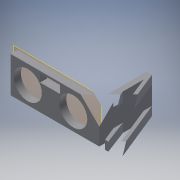
# Autodesk Inventor part: USsensor holder
Saved by Autodesk Inventor 2016 (Build 200138000, 138)
## iProperties
Created: 2018-11-07
Part Number: USsensor holder
Material: Generic
Document SubType Name: Modeling
Designer: anjal
Density: 1 g/cm^3
Appearance: Default
Author: anjal
Autodesk Inventor part; units mm, degrees
ref_plane "YZ Plane" through (0, 0, 0) normal (1, 0, 0) x (0, 1, 0)
ref_plane "XZ Plane" through (0, 0, 0) normal (0, 1, 0) x (-1, 0, 0)
ref_plane "XY Plane" through (0, 0, 0) normal (0, 0, 1) x (1, 0, 0)
ref_plane "Work Plane1" through (7.2648, 18.7113, 1.7167) normal (0, 0, 1) x (1, 0, 0)
sketch "Sketch1" plane through (7.2648, 18.7113, 1.7167) normal (0, 0, 1) x (1, 0, 0)
  circle A0 centre (-12.9413, -0.2667) radius 7.9502 projected
  line L0 (-5.933, 4.5118) -> (5.37, 4.5118) projected
  line L1 (5.37, 9.0584) -> (-5.933, 9.0584) projected
  line L2 (5.37, 9.0584) -> (-5.933, 9.0584) projected
  circle A1 centre (-12.9413, -0.2667) radius 7.9502 projected
  circle A2 centre (12.9413, -0.2667) radius 7.9502 projected
  line L3 (22.7457, -10.1981) -> (22.7457, 10.1981)
  line L4 (22.7457, 10.1981) -> (-22.7457, 10.1981) projected
  line L5 (-22.7457, -10.1981) -> (22.7457, -10.1981)
  line L6 (-22.7457, 10.1981) -> (-22.7457, -10.1981)
  line L7 (-5.933, 6.444) -> (-5.933, 4.5118) projected
  line L8 (-5.933, 9.0584) -> (-5.933, 7.1262) projected
  line L9 (5.37, 4.5118) -> (5.37, 9.0584)
  line L10 (-5.933, 9.0584) -> (-5.933, 4.5118)
  circle A3 centre (-12.9413, -0.2667) radius 8.25
  circle A4 centre (12.9413, -0.2667) radius 8.25
  point P0 (-7.2648, -18.7113)
  dimension "d5" = 16.5
  dimension "d6" = 16.5
  constraints: 10 end point, 3 vertical, 2 centre point, 2 coincident, 1 horizontal, 1 parallel, 3 other
  measures "d5" diameter of A3
  measures "d6" diameter of A4
extrude "Extrusion1" add sketch "Sketch1" along normal blind 4 contours L5 L6 L4 L3 | A3 | A4
sketch "Sketch2" plane through (7.2648, 18.7113, 5.7167) normal (0, 0, 1) x (1, 0, 0)
  line L0 (22.7457, -10.1981) -> (22.7457, 10.1981)
  line L1 (22.7457, 10.1981) -> (27.7457, 10.1981)
  line L2 (27.7457, 10.1981) -> (27.7457, -10.1981)
  line L3 (27.7457, -10.1981) -> (22.7457, -10.1981)
  line L4 (22.7457, -10.1981) -> (22.7457, 10.1981)
  line L5 (24.7457, 10.1981) -> (24.7457, -10.1981)
  point P0 (-7.2648, -18.7113)
  dimension "d7" = 5
  dimension "d8" = 2
  constraints: 12 end point, 2 parallel, 2 perpendicular, 2 point on line, 1 horizontal
  measures "d7" distance of L0.end L1.end
  measures "d8" distance between parallel lines of L0 L5
extrude "Extrusion3" add sketch "Sketch2" against normal blind 30 contours L5 L1 L2 L3
sketch "Sketch3" plane through (7.2648, 18.7113, 5.7167) normal (0, 0, 1) x (1, 0, 0)
  line L0 (22.7457, -10.1981) -> (22.7457, 10.1981) projected
  line L1 (24.7457, -10.1981) -> (24.7457, 10.1981) projected
  line L2 (22.7457, 10.1981) -> (24.7457, 10.1981)
  line L3 (24.7457, 10.1981) -> (24.7457, -10.1981)
  line L4 (24.7457, -10.1981) -> (22.7457, -10.1981)
  line L5 (22.7457, -10.1981) -> (22.7457, 10.1981)
  point P0 (-7.2648, -18.7113)
  constraints: 8 end point, 2 parallel, 1 horizontal, 1 perpendicular
extrude "Extrusion4" add sketch "Sketch3" against normal blind 4
sketch "Sketch4" plane through (-15.4809, 28.9094, 5.7167) normal (0, 1, 0) x (1, 0, 0)
  line L0 (50.4914, 0) -> (50.4914, 30) projected
  line L1 (50.4914, 30) -> (62.668, 0)
  line L2 (62.668, 0) -> (60.736, 0)
  line L3 (60.736, 0) -> (50.4914, 25.24)
  line L4 (55.6137, 0) -> (50.4914, 13.4027)
  line L5 (53.764, 0) -> (50.4914, 8.0628)
  line L6 (50.4914, 13.4027) -> (50.4914, 8.0628)
  line L7 (53.764, 0) -> (55.6137, 0)
  point P0 (15.4809, 5.7167)
  constraints: 14 end point, 5 point on line, 2 parallel, 2 perpendicular, 1 collinear
extrude "Extrusion5" add sketch "Sketch4" against normal blind 5
sketch "Sketch5" plane through (-15.4809, 8.5132, 1.7167) normal (0, -1, 0) x (1, 0, 0)
  line L0 (50.4914, -26) -> (50.4914, -21.24) projected
  line L1 (50.4914, -26) -> (62.668, 4) projected
  line L2 (62.668, 4) -> (60.736, 4) projected
  line L3 (60.736, 4) -> (50.4914, -21.24) projected
  line L4 (50.4914, -9.4027) -> (50.4914, -4.0628) projected
  line L5 (50.4914, -9.4027) -> (55.6137, 4) projected
  line L6 (55.6137, 4) -> (53.764, 4) projected
  line L7 (53.764, 4) -> (50.4914, -4.0628) projected
  point P0 (15.4809, -1.7167)
extrude "Extrusion6" add sketch "Sketch5" against normal blind 5
body "Solid1"
